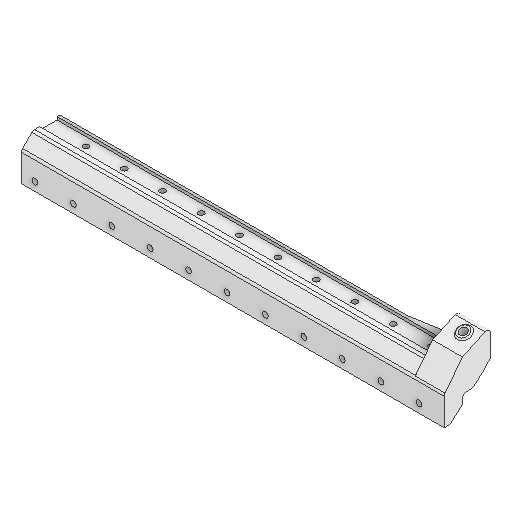
# Autodesk Inventor part: GantryRailMount
Saved by Autodesk Inventor 2026.2 (Build 302298000, 298)
## iProperties
Created: 2026-03-26
Part Number: GantryRailMount
Material: ABS Plastic
Document SubType Name: Modeling
Designer: gaoet
Density: 1.06 g/cm^3
Appearance: Smooth - White
Author: gaoet
Autodesk Inventor part; units mm, degrees
ref_plane "YZ Plane" through (0, 0, 0) normal (1, 0, 0) x (0, 1, 0)
ref_plane "XZ Plane" through (0, 0, 0) normal (0, 1, 0) x (-1, 0, 0)
ref_plane "XY Plane" through (0, 0, 0) normal (0, 0, 1) x (1, 0, 0)
sketch "Sketch1" plane through (0, 0, 0) normal (0, 0, 1) x (1, 0, 0)
  line L0 (-110, -7.5) -> (110, -7.5)
  line L1 (110, -7.5) -> (110, 7.5)
  line L2 (110, 7.5) -> (-110, 7.5)
  line L3 (-110, 7.5) -> (-110, -7.5)
  line L4 (-110, -7.5) -> (110, 7.5) construction
  line L5 (110, -7.5) -> (-110, 7.5) construction
  point P0 (0, 0)
  dimension "d0" = 220
  dimension "d1" = 15
  constraints: 12 end point, 2 midpoint, 2 parallel, 1 horizontal, 1 perpendicular
  measures "d0" distance of L2.end L1.end
  measures "d1" distance of L1.end L0.end
extrude "Extrusion1" add sketch "Sketch1" along normal blind 3
sketch "Sketch2" plane through (0, 0, 3) normal (0, 0, 1) x (1, 0, 0)
  line L0 (110, -7.5) -> (110, 7.5) projected
  line L1 (110, 7.5) -> (-110, 7.5) projected
  line L2 (-110, 7.5) -> (-110, -7.5) projected
  line L3 (-110, -7.5) -> (110, -7.5) projected
  line L4 (-110, -7.5) -> (110, -7.5)
  line L5 (110, -7.5) -> (110, 1.5)
  line L6 (110, 1.5) -> (-110, 1.5)
  line L7 (-110, 1.5) -> (-110, -7.5)
  point P0 (0, 0)
  point P1 (-100, -3)
  point P2 (-110, -3)
  dimension "d4" = 9
  dimension "d5" = 10
  constraints: 8 end point, 2 parallel, 1 horizontal, 1 horizontal alignment, 1 midpoint, 1 perpendicular, 1 point on line
  measures "d4" distance of L5.end L4.end
  measures "d5" distance of point (-110, -3) point (-100, -3)
hole "Hole1" at (-100, -3, 3) direction (0, 0, -1) diameter 3 end through all
pattern_linear "Rectangular Pattern1" count 11 spacing 20 along (1, 0, 0) of "Hole1"
sketch "Sketch3" plane through (110, -7.5, 0) normal (1, 0, 0) x (0, 0, -1)
  line L0 (0, 0) -> (0, 15) projected
  line L1 (0, 15) -> (-3, 15) projected
  line L2 (-3, 0) -> (-3, 15) projected
  line L3 (0, 0) -> (-3, 0) projected
  line L4 (-3, 15) -> (17, 15)
  line L5 (17, 15) -> (17, 21)
  line L6 (17, 21) -> (-3, 21)
  line L7 (-3, 21) -> (-3, 15)
  line L8 (0, 15) -> (1.5, 15)
  line L9 (1.5, 15) -> (1.5, 9)
  line L10 (1.5, 9) -> (0, 9)
  line L11 (0, 9) -> (0, 15)
  point P0 (0, 7.5)
  point P1 (0, 9)
  dimension "d16" = 20
  dimension "d17" = 6
  dimension "d18" = 1.5
  dimension "d19" = 6
  constraints: 16 end point, 4 parallel, 2 horizontal, 2 perpendicular
  measures "d16" distance of L1.end L4.end
  measures "d17" distance of L6.end L1.end
  measures "d18" distance of L9.end L10.end
  measures "d19" distance of L8.end L9.end
extrude "Extrusion2" add sketch "Sketch3" against normal up to surface (220 mm away) contours L0 L4 L9 L10 | L1 L7 L6 L5 L4
sketch "Sketch4" plane through (110, -7.5, 3) normal (1, 0, 0) x (0, 0, -1)
  line L0 (3, 0) -> (3, 9) projected
  line L1 (3, 9) -> (4.5, 9) projected
  line L2 (4.5, 9) -> (4.5, 15) projected
  line L3 (4.5, 15) -> (20, 15) projected
  line L4 (20, 15) -> (20, 21) projected
  line L5 (20, 21) -> (0, 21) projected
  line L6 (0, 0) -> (0, 21) projected
  line L7 (3, 0) -> (0, 0) projected
  line L8 (3, 0) -> (20, 15)
  line L9 (9.5, 5.7353) -> (9.5, 10.5)
  line L10 (9.5, 10.5) -> (14.9, 10.5)
  point P0 (3, 7.5)
  point P1 (9.5, 8.1176)
  dimension "d48" = 9.5
  dimension "d49" = 4.5
  constraints: 6 end point, 2 point on line, 1 midpoint, 1 perpendicular, 1 vertical
  measures "d48" distance from line of L6 point (9.5, 8.118)
  measures "d49" distance between parallel lines of L3 L10
extrude "Extrusion3" add sketch "Sketch4" along normal blind 3 contours L7 L6 L5 L4 L3 L2 L1 L0 | L0 L1 L2 L3 L8 L10 L9
sketch "Sketch5" plane through (-110, -7.5, 0) normal (-1, 0, 0) x (0, 0, 1)
  line L0 (0, 9) -> (0, 0) projected
  line L1 (0, 0) -> (3, 0) projected
  line L2 (3, 21) -> (3, 0) projected
  line L3 (-17, 21) -> (3, 21) projected
  line L4 (-17, 15) -> (-17, 21) projected
  line L5 (-1.5, 15) -> (-17, 15) projected
  line L6 (-1.5, 9) -> (-1.5, 15) projected
  line L7 (0, 9) -> (-1.5, 9) projected
  point P0 (0, 7.5)
extrude "Extrusion4" cut sketch "Sketch5" against normal blind 3
sketch "Sketch6" plane through (113, 13.5, 3) normal (0, 1, 0) x (1, 0, 0)
  line L0 (-220, 20) -> (-220, 0) projected
  line L1 (-220, 0) -> (0, 0) projected
  line L2 (0, 20) -> (0, 0) projected
  line L3 (0, 20) -> (-220, 20) projected
  point P0 (-113, 3)
  point P1 (-20.5, 14)
  dimension "d26" = 20.5
  dimension "d27" = 6
  measures "d26" distance from line of L2 point (-20.5, 14)
  measures "d27" distance from line of L3 point (-20.5, 14)
hole "Hole2" at (92.5, 13.5, -11) direction (0, -1, 0) diameter 3 end through all
pattern_linear "Rectangular Pattern2" count 10 spacing 20 along (-1, 0, 0) of "Hole2"
sketch "Sketch7" plane through (113, 13.5, 3) normal (0, 1, 0) x (1, 0, 0)
  circle A0 centre (-200.5, 14) radius 1.5 projected
  circle A1 centre (-180.5, 14) radius 1.5 projected
  circle A2 centre (-160.5, 14) radius 1.5 projected
  circle A3 centre (-140.5, 14) radius 1.5 projected
  circle A4 centre (-120.5, 14) radius 1.5 projected
  circle A5 centre (-100.5, 14) radius 1.5 projected
  circle A6 centre (-80.5, 14) radius 1.5 projected
  circle A7 centre (-60.5, 14) radius 1.5 projected
  circle A8 centre (-40.5, 14) radius 1.5 projected
  circle A9 centre (-20.5, 14) radius 1.5 projected
  line L0 (-220, 20) -> (-220, 0) projected
  line L1 (-220, 0) -> (0, 0) projected
  line L2 (0, 20) -> (0, 0) projected
  line L3 (0, 20) -> (-220, 20) projected
  line L4 (-220, 9.5) -> (-10.5, 9.5)
  line L5 (-10.5, 9.5) -> (-10.5, 20)
  line L6 (-10.5, 20) -> (-220, 20)
  line L7 (-220, 20) -> (-220, 9.5)
  line L8 (-10.5, 9.5) -> (0, 9.5)
  point P0 (-113, 3)
  dimension "d38" = 10.5
  dimension "d39" = 10
  constraints: 10 end point, 3 point on line, 2 horizontal, 2 parallel, 1 perpendicular
  measures "d38" distance between parallel lines of L6 L4
  measures "d39" distance from line of A9.centre L5
extrude "Extrusion5" cut sketch "Sketch7" against normal blind 1.5 contours L3 L5 L4 L0 | L3 L2 L8 L5
sketch "Sketch8" plane through (110, 7.5, -17) normal (0, -1, 0) x (1, 0, 0)
  circle A0 centre (-197.5, 6) radius 1.5 projected
  circle A1 centre (-177.5, 6) radius 1.5 projected
  circle A2 centre (-157.5, 6) radius 1.5 projected
  circle A3 centre (-137.5, 6) radius 1.5 projected
  circle A4 centre (-117.5, 6) radius 1.5 projected
  circle A5 centre (-97.5, 6) radius 1.5 projected
  circle A6 centre (-77.5, 6) radius 1.5 projected
  circle A7 centre (-57.5, 6) radius 1.5 projected
  circle A8 centre (-37.5, 6) radius 1.5 projected
  circle A9 centre (-17.5, 6) radius 1.5 projected
  line L0 (-217, 15.5) -> (-217, 0) projected
  line L1 (0, 0) -> (-217, 0) projected
  line L2 (0, 15.5) -> (0, 0) projected
  line L3 (0, 15.5) -> (-217, 15.5) projected
  line L4 (-19.0877, 3.25) -> (-20.6754, 6)
  line L5 (-20.6754, 6) -> (-19.0877, 8.75)
  line L6 (-19.0877, 8.75) -> (-15.9123, 8.75)
  line L7 (-15.9123, 8.75) -> (-14.3246, 6)
  line L8 (-14.3246, 6) -> (-15.9123, 3.25)
  line L9 (-15.9123, 3.25) -> (-19.0877, 3.25)
  point P0 (-110, 17)
  dimension "d42" = 5.5
  constraints: 12 end point, 1 coincident, 1 horizontal, 13 other
  measures "d42" distance between parallel lines of L6 L9
extrude "Extrusion6" cut sketch "Sketch8" against normal blind 2.4 contours L4 L5 L6 L7 L8 L9
pattern_linear "Rectangular Pattern3" count 10 spacing 20 along (-1, 0, 0) of "Extrusion6"
fillet "Fillet1" radius 2 3 edges at (111.5, -1.7647, -6.5) (111.5, 3, -11.9) (111.5, 3, -6.5)
chamfer "Chamfer2" distance 5 distance2 8 1 edges at (110, 7.5, -9.25) measured on face at (110, 7, -9.25)
chamfer "Chamfer3" distance 6 angle 45 1 edges at (3, 13.5, 3)
fillet "Fillet2" radius 2 2 edges at (3, 13.5, -3) (3, 7.5, 3)
sketch "Sketch10" plane through (113, -7.5, 3) normal (1, 0, 0) x (0, 0, -1)
  arc A0 (0.5858, 15.5858) -> (0, 14.1716) centre (2, 14.1716) ccw projected
  line L0 (0, 14.1716) -> (0, 0) projected
  line L1 (0, 0) -> (3, 0) projected
  line L2 (3, 0) -> (8.8232, 5.1382) projected
  arc A1 (8.8232, 5.1382) -> (9.5, 6.6378) centre (7.5, 6.6378) ccw projected
  line L3 (9.5, 6.6378) -> (9.5, 8.5) projected
  arc A2 (11.5, 10.5) -> (9.5, 8.5) centre (11.5, 8.5) ccw projected
  line L4 (11.5, 10.5) -> (14.1438, 10.5) projected
  arc A3 (14.1438, 10.5) -> (15.467, 11.0003) centre (14.1438, 12.5) ccw projected
  line L5 (15.467, 11.0003) -> (20, 15) projected
  line L6 (20, 15) -> (20, 19.5) projected
  line L7 (20, 19.5) -> (9.5, 19.5) projected
  line L8 (9.5, 19.5) -> (9.5, 21) projected
  line L9 (9.5, 21) -> (6.8284, 21) projected
  arc A4 (6.8284, 21) -> (5.4142, 20.4142) centre (6.8284, 19) ccw projected
  line L10 (0.5858, 15.5858) -> (5.4142, 20.4142) projected
  line L11 (9.5, 21) -> (9.5, 27.1369)
  line L12 (9.5, 27.1369) -> (24.11, 33.9496)
  line L13 (24.11, 33.9496) -> (24.11, 19.5)
  line L14 (24.11, 19.5) -> (20, 19.5)
  line L15 (24.11, 19.5) -> (20, 15)
  line L16 (9.5, 27.1369) -> (0.418, 15.3952)
  arc A5 (0.5858, 15.5858) -> (0, 14.1716) centre (2, 14.1716) ccw projected
  line L17 (9, 34) -> (22, 34) construction
  line L18 (22, 34) -> (22, 38) construction
  line L19 (22, 38) -> (9, 38) construction
  line L20 (9, 38) -> (9, 34) construction
  line L21 (9, 34) -> (22, 38) construction
  line L22 (22, 34) -> (9, 38) construction
  circle A6 centre (22, 36) radius 1 construction
  line L23 (22.8452, 34.1874) -> (11.0632, 28.6933) construction
  line L24 (11.0632, 28.6933) -> (9.3728, 32.3186) construction
  line L25 (9.3728, 32.3186) -> (21.1548, 37.8126) construction
  line L26 (21.1548, 37.8126) -> (22.8452, 34.1874) construction
  line L27 (22.8452, 34.1874) -> (9.3728, 32.3186) construction
  line L28 (11.0632, 28.6933) -> (21.1548, 37.8126) construction
  circle A7 centre (22, 36) radius 1 construction
  point P0 (3, 7.5)
  point P1 (15.5, 36)
  point P2 (16.109, 33.253)
  dimension "d62" = 4.11
  dimension "d63" = 25
  dimension "d74" = 13
  dimension "d75" = 4
  dimension "d76" = 15.5
  dimension "d77" = 34
  dimension "d78" = 2
  dimension "d79" = 4
  dimension "d80" = 0.75
  constraints: 36 end point, 6 midpoint, 6 parallel, 3 perpendicular, 2 centre point, 1 concentric, 1 equal length, 1 horizontal, 1 point on circle, 1 tangent, 1 vertical
  measures "d62" distance between parallel lines of L13 L6
  measures "d63" angle of L7 L12
  measures "d74" distance of L19.end L18.end
  measures "d75" distance of L18.end L17.end
  measures "d76" distance from line of L0 point (15.5, 36)
  measures "d77" distance between parallel lines of L1 L17
  measures "d78" diameter of A6
  measures "d79" distance of L23.end L24.end
  measures "d80" distance between parallel lines of L12 L23
extrude "Extrusion7" add sketch "Sketch10" against normal blind 15.5 contours A0 L16 L11 L9 A4 L10 | L12 L13 L14 L7 L8 L11 | L15 L6 L14
fillet "Fillet3" radius 2 1 edges at (105.25, 26.4496, -21.11)
chamfer "Chamfer4" distance 4.11 angle 80 1 edges at (97.5, 9.75, -17) measured on face at (97.5, 9.75, -17.5)
sketch "Sketch11" plane through (113, 12, 3) normal (0, 1, 0) x (1, 0, 0)
  line L0 (-15.5, 9.5) -> (-15.5, 24.11) projected
  line L1 (-38.8087, 20) -> (-15.5, 24.11) projected
  line L2 (-220, 20) -> (-38.8087, 20) projected
  line L3 (-220, 9.5) -> (-220, 20) projected
  line L4 (-15.5, 9.5) -> (-220, 9.5) projected
  circle A0 centre (-20.5, 14) radius 1.5 projected
  circle A1 centre (-60.5, 14) radius 1.5 projected
  circle A2 centre (-80.5, 14) radius 1.5 projected
  circle A3 centre (-100.5, 14) radius 1.5 projected
  circle A4 centre (-120.5, 14) radius 1.5 projected
  circle A5 centre (-140.5, 14) radius 1.5 projected
  circle A6 centre (-160.5, 14) radius 1.5 projected
  circle A7 centre (-180.5, 14) radius 1.5 projected
  circle A8 centre (-200.5, 14) radius 1.5 projected
  circle A9 centre (-40.5, 14) radius 1.5 projected
  line L5 (-220, 18.5) -> (-15.5, 18.5)
  point P0 (-113, 3)
  dimension "d71" = 9
  constraints: 2 end point, 2 point on line, 1 perpendicular
  measures "d71" distance between parallel lines of L4 L5
extrude "Extrusion8" add sketch "Sketch11" along normal blind 1.5 contours L5 L3 L2 L1 L0
sketch "Sketch12" plane through (97.5, 19.6369, -6.5) normal (0, 0.9063078, 0.4226183) x (1, 0, 0)
  line L0 (0, 12.981) -> (15.5, 12.981) projected
  line L1 (0, 0) -> (0, 12.981) projected
  line L2 (15.5, 0) -> (0, 0) projected
  line L3 (15.5, 12.981) -> (15.5, 0) projected
  line L4 (15.5, 15.0746) -> (15.5, 2.0746) construction
  point P0 (-97.5, -14.1899)
  point P1 (8.5, 8.5746)
  point P2 (15.5, 8.5746)
  dimension "d81" = 7
  constraints: 1 horizontal alignment
  measures "d81" distance from line of L3 point (8.5, 8.575)
hole "Hole3" at (106, 23.2606, -14.2712) direction (0, -0.9063078, -0.4226183) diameter 4 depth 11
sketch "Sketch13" plane through (97.5, 19.6369, -6.5) normal (0, 0.9063078, 0.4226183) x (1, 0, 0)
  circle A0 centre (8.5, 8.5746) radius 2 projected
  line L0 (0, 12.981) -> (15.5, 12.981) projected
  line L1 (0, 0) -> (0, 12.981) projected
  line L2 (15.5, 0) -> (0, 0) projected
  line L3 (15.5, 12.981) -> (15.5, 0) projected
  circle A1 centre (8.5, 8.5746) radius 3
  point P0 (-97.5, -14.1899)
  dimension "d89" = 1
  constraints: 1 centre point
  measures "d89" radial gap between concentric circles of A0 A1
extrude "Extrusion9" add sketch "Sketch13" along normal blind 0.75 contours A1
chamfer "Chamfer5" distance 0.75 angle 45 1 edges at (103, 23.2606, -14.2712)
sketch "Sketch14" plane through (110, -7.5, 3) normal (-1, 0, 0) x (0, 0, 1)
  line L0 (-10.1771, 10) -> (-4.5, 10) projected
  arc A0 (-9.5, 8.5) -> (-10.1771, 10) centre (-11.5, 8.5) ccw projected
  line L1 (-9.5, 6.6378) -> (-9.5, 8.5) projected
  arc A1 (-9.5, 6.6378) -> (-8.8232, 5.1382) centre (-7.5, 6.6378) ccw projected
  line L2 (-3, 0) -> (-8.8232, 5.1382) projected
  line L3 (-3, 0) -> (-3, 9) projected
  line L4 (-3, 9) -> (-4.5, 9) projected
  line L5 (-4.5, 9) -> (-4.5, 10) projected
  line L6 (-9.5, 8.5) -> (-9.5, 10)
  point P0 (-3, 7.5)
  constraints: 2 end point, 1 point on line, 1 vertical
extrude "Extrusion10" add sketch "Sketch14" along normal blind 5 contours L0 L5 L4 L3 L2 A1 L1 L6
sketch "Sketch15" plane through (113, 1, -6.5) normal (0, 0, -1) x (-1, 0, 0)
  line L0 (0, 0) -> (3, 0) projected
  line L1 (0, -1.8622) -> (0, 0) projected
  line L2 (0, -1.8622) -> (8, -1.8622) projected
  line L3 (8, 1.5) -> (8, -1.8622) projected
  line L4 (3, 1.5) -> (8, 1.5) projected
  line L5 (3, 0) -> (3, 1.5) projected
  line L6 (0, 6.5) -> (0, 11) projected
  line L7 (11, 6.5) -> (0, 6.5) projected
  line L8 (11, 6.5) -> (38.8087, 6.5) projected
  line L9 (38.8087, 6.5) -> (15.5, 11) projected
  line L10 (15.5, 11) -> (15.5, 11) projected
  line L11 (0, 11) -> (15.5, 11) projected
  line L12 (8, 1.5) -> (16, 6.5)
  line L13 (11, 6.5) -> (4.6005, 2.5003) projected
  line L14 (3, 1.5) -> (3.8, 2) projected
  line L15 (11, 6.5) -> (3, 1.5) projected
  line L16 (11, 6.5) -> (4.6005, 2.5003) projected
  line L17 (3.8, 2) -> (4.6005, 2.5003) projected
  point P0 (113, -1)
  constraints: 2 end point, 1 parallel, 1 point on line
extrude "Extrusion11" add sketch "Sketch15" against normal up to surface (5 mm away) contours L14 L15 L13 L8 L12 L4
fillet "Fillet4" radius 2 2 edges at (105, 2.5, -4) (97, 7.5, -4)
body "Solid1"
